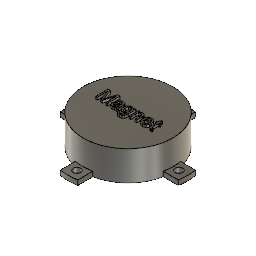
cap v4 (Autodesk Fusion 360 design; units mm, degrees)
Autodesk Fusion 360 part; units mm, degrees
sketch "Sketch1" plane through (0, 0, 0) normal (0, 0, 1) x (1, 0, 0)
  circle A0 centre (0, 0) radius 16
  circle A1 centre (0, 0) radius 18
  dimension "d1" = 32
  dimension "d2" = 2
  constraint coincident A0.centre A1.centre
  constraint concentric A0 A1
  measures "d1" diameter of A0
  measures "d2" distance of A0 A1
extrude "Extrude1" add sketch "Sketch1" along normal blind 10
sketch "Sketch2" plane through (0, 0, 10) normal (0, 0, 1) x (-1, 0, 0)
  circle A0 centre (0, 0) radius 16
  circle A1 centre (0, 0) radius 18
  circle A2 centre (0, 0) radius 18
  constraint coincident A0.centre A1.centre
  constraint tangent A1 A2
extrude "Extrude2" add sketch "Sketch2" along normal blind 2 contours A0 | A1 A2
sketch "Sketch3" plane through (0, 0, 0) normal (0, 0, -1) x (1, 0, 0)
  circle A0 centre (0, 0) radius 16
  circle A1 centre (0, 0) radius 18
  line L0 (-3.5, 24) -> (3.5, 24)
  line L1 (3.5, 24) -> (3.5, -27)
  line L2 (3.5, -27) -> (-3.5, -27)
  line L3 (-3.5, -27) -> (-3.5, 24)
  line L4 (0, 0) -> (0, 18)
  line L5 (0, 18) -> (0, 24)
  circle A2 centre (0, 20.5) radius 1.5
  line L6 (0, 19) -> (0.9, 19)
  circle A3 centre (0, 0) radius 24
  line L7 (27, -3.5) -> (-24, -3.5)
  line L8 (-24, 3.5) -> (27, 3.5)
  circle A4 centre (-20.5, 0) radius 1.5
  line L9 (3.5, 27) -> (3.5, -24)
  line L10 (-3.5, -24) -> (-3.5, 27)
  circle A5 centre (0, -20.5) radius 1.5
  line L11 (-27, 3.5) -> (24, 3.5)
  line L12 (24, -3.5) -> (-27, -3.5)
  circle A6 centre (20.5, 0) radius 1.5
  dimension "d7" = 7
  dimension "d8" = 90
  dimension "d9" = 3
  dimension "d10" = 1
  dimension "d11" = 3.5
  dimension "d13" = 360
  constraint horizontal L0
  constraint vertical L1
  constraint horizontal L2
  constraint vertical L3
  constraint coincident A0.centre A1.centre
  constraint coincident A1 L4.end
  constraint parallel L1 L4
  constraint midpoint L0 L5.end
  constraint coincident L5 A2.centre
  constraint coincident A2 L6.start
  constraint coincident L5 L6.start
  constraint tangent A2 L6
  constraint coincident L5.end A3
  measures "d7" distance of L0.start L0.end
  measures "d8" angle of L0 L5
  measures "d9" diameter of A2
  measures "d10" distance of L4.end L6.start
  measures "d11" distance of L0 A2.centre
extrude "Extrude3" add sketch "Sketch3" against normal blind 3 contours A1 A3 L7 L8 L11 L12 | A1 L1 L5 A2 A3 L9 | A1 L1 L3 A3 L9 L10 | A1 L3 L5 A2 A3 L10 | A1 A3 L7 L8 L11 L12
extrude "Extrude4" cut 4 faces at (2.8333, -20.6333, 3) (-20.6707, 2.8319, 3) (20.6707, -2.8319, 3) (-2.8333, 20.6333, 3) along direction (0, 0, -1) blind 1
sketch "Sketch4" plane through (0, 0, 12) normal (0, 0, 1) x (-1, 0, 0)
  circle A0 centre (0, 0) radius 18
  line L0 (11, 2) -> (-11, 2) construction
  line L1 (-11, 2) -> (-11, -3) construction
  line L2 (-11, -3) -> (11, -3) construction
  line L3 (11, -3) -> (11, 2) construction
  dimension "d18" = 5
  text T0 "Magnet" font "Arial" height 5 align left top in box 22 x 5 at (11, 2) x (-1, 0) y (0, -1) spacing 1 kerned
extrude "Extrude5" add sketch "Sketch4" along normal blind 1 text T0
